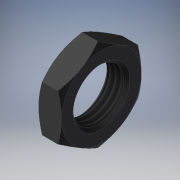
# Autodesk Inventor part: SNJ-016C
Saved by Autodesk Inventor 2019 (Build 230136000, 136)
## iProperties
Created: 2024-03-16
Part Number: SNJ-016C
Material: Generic
Catalog Web Link: www.cadenas.de
Description: CJ2-Z_SNJ-Mounting Nut
Vendor: SMC
Document SubType Name: Modeling
Designer: psAdmin
Manufacturer: SMC
Mass: 0.414663 g
Surface Area: 4.87707 cm^2
Volume: 0.414663 cm^3
Density: 1 g/cm^3
Appearance: PSOLRGB-191-191-191
Category: PARTsolutions
Company: SMC
Title: SNJ-016C
Author: Cadenas PARTsolutions
Comments: Mounting Nut
PSOL_IDENT_0: {$CADENAS_DATA/23d-libs/smc_jp/actuator/standard_air_cylinder/cj2/accessories/cj2_z_snj.prj},159 {VT
PSOL_IDENT_1: YP=3D},{NB=SNJ-016C},{LINA=SNJ-016C},{NN=CJ2-Z_SNJ},{DATE=07.03.2024 03:01:46},{GEOMDATE=12.05.2020
PSOL_IDENT_2: 08:15:39},{VERSION=},{LINEID=30},{WBVAR=},{WBNUMERIC=}  {NB=SNJ-016C},{LINA=SNJ-016C},{KT=DUMMY},{MO
PSOL_IDENT_3: DEL=SNJ-016C},{BORE=16},{B1=14},{C1=16.2},{D=M10x1.0},{D1=10},{D2=1},{H1=4},{ORDER=SNJ-016C}
NB: SNJ-016C
NN: CJ2-Z_SNJ
NT: Mounting Nut
NBSYN: $MODEL.
LINA: SNJ-016C
CATALOG: SMC (JP
MODEL: SNJ-016C
BORE: 16
B1: 14
C1: 16.2
D: M10x1.0
H1: 4
SUPPLIER: SMC
ARTICLENO: SNJ-016C
BOMINFO: SNJ-016C
CREATOR: CADENAS GmbH
Autodesk Inventor part; units mm, degrees
sketch "B" plane through (0, 0, 0) normal (1, 0, 0) x (0, 1, 0)
  line L0 (-4.0415, 7) -> (-8.0829, 0)
  line L1 (-8.0829, 0) -> (-4.0415, -7)
  line L2 (-4.0415, -7) -> (4.0415, -7)
  line L3 (4.0415, -7) -> (8.0829, 0)
  line L4 (8.0829, 0) -> (4.0415, 7)
  line L5 (4.0415, 7) -> (-4.0415, 7)
  constraints: 12 end point
extrude "Extrusion1" add sketch "B" along normal mid plane 4
sketch "Sketch_2" plane through (0, 0, 0) normal (0, 0, 1) x (1, 0, 0)
  line L0 (2, 0) -> (-2, 0)
  line L1 (-2, 0) -> (-2, 5)
  line L2 (-2, 5) -> (-1.4585, 4.4585)
  line L3 (-1.4585, 4.4585) -> (1.4585, 4.4585)
  line L4 (1.4585, 4.4585) -> (2, 5)
  line L5 (2, 5) -> (2, 0)
  line L6 (2, 0) -> (-2, 0)
  constraints: 14 end point
revolve "Revolution1" cut sketch "Sketch_2" angle 360 about axis through (2, 0, 0) along (1, 0, 0)
thread "Thread1" size "M10x1" class "6H" standard "ISO Metric profile" full length
sketch "Sketch_3" plane through (0, 0, 0) normal (0, 0, 1) x (1, 0, 0)
  line L0 (50, 0) -> (-50, 0)
  line L1 (-7, 1) -> (-2, 1)
  line L2 (-2, 1) -> (-2, 7)
  line L3 (-2, 7) -> (0, 10.4641)
  line L4 (0, 10.4641) -> (2, 7)
  line L5 (2, 7) -> (2, 1)
  line L6 (2, 1) -> (7, 1)
  line L7 (7, 1) -> (7, 17)
  line L8 (7, 17) -> (-7, 17)
  line L9 (-7, 17) -> (-7, 1)
  constraints: 20 end point
revolve "Revolution2" cut sketch "Sketch_3" angle 360 about axis through (50, 0, 0) along (1, 0, 0)
ref_plane "nt_XY" through (0, 0, 0) normal (1, 0, 0) x (0, 0, -1)
ref_plane "nt_YZ" through (0, 0, 0) normal (0, 0, -1) x (0, 1, 0)
ref_plane "nt_ZX" through (0, 0, 0) normal (0, 1, 0) x (1, 0, 0)
ref_plane "ntj_XY" through (2, 0, 0) normal (1, 0, 0) x (0, 0, -1)
ref_plane "ntj_YZ" through (2, 0, 0) normal (0, 0, -1) x (0, 1, 0)
ref_plane "ntj_ZX" through (2, 0, 0) normal (0, 1, 0) x (1, 0, 0)
body "Solid1"
